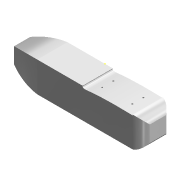
# Autodesk Inventor part: body
Saved by Autodesk Inventor 2020 (Build 240168000, 168)
## iProperties
Part Number: body
Material: Generic
Document SubType Name: Modeling
Designer: alifhabib
Appearance: Default
Author: alifhabib
Autodesk Inventor part; units mm, degrees
ref_plane "YZ Plane" through (0, 0, 0) normal (1, 0, 0) x (0, 1, 0)
ref_plane "XY Plane" through (0, 0, 0) normal (0, 0, 1) x (1, 0, 0)
sketch "Sketch1" plane through (0, 0, 0) normal (0, 0, 1) x (1, 0, 0)
  line L0 (-337.5, 75) -> (337.5, 75)
  line L1 (337.5, 75) -> (337.5, -75)
  line L2 (337.5, -75) -> (-337.5, -75)
  line L3 (-337.5, -75) -> (-337.5, 75)
  line L4 (-337.5, 75) -> (337.5, -75) construction
  line L5 (337.5, 75) -> (-337.5, -75) construction
  point P0 (0, 0)
  dimension "d0" = 675
  dimension "d1" = 150
  constraints: 12 end point, 2 midpoint, 2 parallel, 1 horizontal, 1 perpendicular
  measures "d0" distance of L1.end L2.end
  measures "d1" distance of L0.end L1.end
extrude "Extrusion1" add sketch "Sketch1" along normal blind 150
sketch "Sketch2" plane through (0, 0, 150) normal (0, 0, 1) x (1, 0, 0)
  line L0 (-400, 225) -> (400, 225)
  line L1 (400, 225) -> (400, -225)
  line L2 (400, -225) -> (-400, -225)
  line L3 (-400, -225) -> (-400, 225)
  line L4 (-337.5, 0) -> (-187.5, 0)
  line L5 (-337.5, 0) -> (-337.5, 40)
  line L6 (-337.5, 0) -> (-337.5, -40)
  line L7 (337.5, 0) -> (287.5, 0)
  line L8 (337.5, 0) -> (337.5, 40)
  line L9 (337.5, 0) -> (337.5, -40)
  arc A0 (-187.5, 75) -> (-337.5, 40) centre (-150.241, -423.6098) ccw
  line L10 (-187.5, 75) -> (287.5, 75)
  arc A1 (337.5, 40) -> (287.5, 75) centre (273.2116, 1.3736) ccw
  arc A2 (-337.5, -40) -> (-187.5, -75) centre (-150.241, 423.6098) ccw
  line L11 (-187.5, -75) -> (287.5, -75)
  arc A3 (287.5, -75) -> (337.5, -40) centre (273.2116, -1.3736) ccw
  point P0 (0, 0)
  dimension "d4" = 800
  dimension "d5" = 450
  dimension "d14" = 50
  dimension "d15" = 40
  dimension "d16" = 40
  dimension "d17" = 500
  dimension "d18" = 75
  constraints: 24 end point, 8 point on circle, 4 centre point, 4 symmetric about line, 3 horizontal, 2 parallel, 1 perpendicular, 2 other
  measures "d4" distance of L1.end L2.end
  measures "d5" distance of L0.end L1.end
  measures "d14" distance of L7.start L7.end
  measures "d15" distance of L7.start L8.end
  measures "d16" distance of L7.start L9.end
  measures "d17" radius of A0
  measures "d18" radius of A1
extrude "Extrusion2" cut sketch "Sketch2" against normal blind 150
sketch "Sketch3" plane through (-187.5, 75, 0) normal (0, 1, 0) x (1, 0, 0)
  line L0 (-312.5, 400) -> (687.5, 400)
  line L1 (687.5, 400) -> (687.5, -400)
  line L2 (687.5, -400) -> (-312.5, -400)
  line L3 (-312.5, -400) -> (-312.5, 400)
  line L4 (525, 0) -> (525, -150) projected
  line L5 (525, -75) -> (475, -75)
  line L6 (-150, -150) -> (-150, 0) projected
  line L7 (-150, -75) -> (-150, -35)
  line L8 (0, 0) -> (475, 0) projected
  arc A0 (0, 0) -> (-150, -35) centre (37.259, -498.6098) ccw
  line L9 (525, -75) -> (525, -35)
  line L10 (525, 0) -> (475, 0) projected
  arc A1 (525, -35) -> (475, 0) centre (460.7116, -73.6264) ccw
  line L11 (-150, -75) -> (-150, -115)
  arc A2 (-150, -115) -> (0, -150) centre (37.259, 348.6098) ccw
  line L12 (525, -75) -> (525, -115)
  arc A3 (475, -150) -> (525, -115) centre (460.7116, -76.3736) ccw
  line L13 (475, -150) -> (0, -150) projected
  line L14 (0, -150) -> (475, -150)
  point P0 (187.5, 0)
  dimension "d23" = 40
  dimension "d24" = 500
  dimension "d25" = 40
  dimension "d26" = 75
  constraints: 20 end point, 8 point on circle, 4 centre point, 2 horizontal, 2 midpoint, 2 parallel, 2 point on line, 1 perpendicular
  measures "d23" distance of L7.start L7.end
  measures "d24" radius of A0
  measures "d25" distance of L5.start L9.end
  measures "d26" radius of A1
extrude "Extrusion3" cut sketch "Sketch3" against normal blind 150 contours L0 L1 L2 L3 | L4 A1 L10
sketch "Sketch4" plane through (0, 0, 150) normal (0, 0, 1) x (1, 0, 0)
  spline S0 degree 4 poles (287.5, 72) (275.7106, 75.6696) (272.2633, 78.0977) (241.0041, 87.3899) (212.1922, 94.1056) (186.8012, 99.4436) (162.2405, 102.6617) (136.499, 103.3609) (115.3024, 103.9082) (87.5125, 99.0497) (77.8593, 96.7101) (62.5936, 91.6603) (56.4872, 88.8369) (50.2371, 85.9481) (43.0983, 79.8721) (41.263, 78.3038) (35.0709, 71.8313) (41.0621, 66.1136) (43.5349, 66.5804) (51.0426, 65.1949) (57.2037, 65.9223) (63.437, 66.335) (78.7454, 67.9836) (88.3716, 68.7088) (116.236, 70.8678) (137.1854, 71.569) (162.8258, 72.2403) (187.1936, 73.1117) (212.5281, 72.7462) (241.0177, 72.4966) (272.1667, 71.6209) (275.8592, 71.8531) (287.5, 71.2) knots 0 0 0 0 0 0.082908 0.121264 0.162409 0.203325 0.244067 0.284728 0.322462 0.357388 0.387441 0.412707 0.436373 0.45684 0.477222 0.496964 0.514702 0.533384 0.551956 0.570848 0.593257 0.617753 0.647324 0.681959 0.719554 0.76011 0.800663 0.841217 0.881776 0.91937 1 1 1 1 1
  arc A0 (287.5, 71.2) -> (287.5, 72) centre (286.5835, 71.6) ccw
  point P0 (0, 0)
  point P1 (274.89, 76.355)
  point P2 (262.2875, 80.71)
  point P3 (237.1175, 87.97)
  point P4 (211.975, 94.0325)
  point P5 (186.8575, 99.02)
  point P6 (161.785, 102.1575)
  point P7 (136.7575, 103.3225)
  point P8 (111.775, 102.5875)
  point P9 (86.8675, 98.68)
  point P10 (74.4425, 95.465)
  point P11 (62.0425, 91.2)
  point P12 (55.855, 88.53)
  point P13 (49.685, 85.06)
  point P14 (43.5475, 80.2425)
  point P15 (40.49, 77.395)
  point P16 (37.5, 71.6)
  point P17 (40.73, 67.15)
  point P18 (43.875, 66.3)
  point P19 (50.14, 65.645)
  point P20 (56.385, 65.7925)
  point P21 (62.6225, 66.3375)
  point P22 (75.095, 67.555)
  point P23 (87.57, 68.6475)
  point P24 (112.5275, 70.43)
  point P25 (137.5025, 71.54)
  point P26 (162.485, 72.275)
  point P27 (187.47, 72.86)
  point P28 (212.4725, 72.77)
  point P29 (237.48, 72.43)
  point P30 (262.4925, 71.94)
  point P31 (274.9975, 71.7075)
  point P32 (287.5, 75)
  dimension "d31" = 1
  constraints: 2 point on circle, 1 centre point, 33 other
  measures "d31" radius of A0
extrude "Extrusion4" cut sketch "Sketch4" against normal blind 150
sketch "Sketch5" plane through (0, 0, 150) normal (0, 0, 1) x (1, 0, 0)
  spline S0 degree 4 poles (278.5919, 75) (280.4602, 74.3245) (282.4435, 73.6259) (284.707, 72.8694) (287.5, 72) knots 0 0 0 0 0 1 1 1 1 1 projected
  line L0 (287.5, 72) -> (287.5, 75) projected
  line L1 (287.5, 75) -> (278.5919, 75) projected
  point P0 (0, 0)
  constraints: 1 other
extrude "Extrusion5" cut sketch "Sketch5" against normal blind 150
sketch "Sketch8" plane through (0, 0, 150) normal (0, 0, 1) x (1, 0, 0)
  line L0 (38.5386, 75) -> (-187.5, 75) projected
  line L1 (-187.5, 75) -> (-187.5, -75) projected
  line L2 (-187.5, -75) -> (287.5, -75) projected
  line L3 (287.5, -75) -> (287.5, 71.2) projected
  arc A0 (-337.5, -40) -> (-187.5, -75) centre (-150.241, 423.6098) ccw projected
  line L4 (-187.5, 75) -> (-187.5, -75) projected
  arc A1 (-187.5, 75) -> (-337.5, 40) centre (-150.241, -423.6098) ccw projected
  line L5 (-337.5, -40) -> (-337.5, 40) projected
  line L6 (287.5, -75) -> (287.5, 71.2) projected
  arc A2 (287.5, -75) -> (337.5, -40) centre (273.2116, -1.3736) ccw projected
  line L7 (337.5, 40) -> (337.5, -40) projected
  arc A3 (337.5, 40) -> (287.5, 75) centre (273.2116, 1.3736) ccw projected
  line L8 (287.5, 72) -> (287.5, 75) projected
  point P0 (0, 0)
  constraints: 1 vertical alignment, 1 other
sketch "Sketch9" plane through (-187.5, 75, 150) normal (0, 1, 0) x (1, 0, 0)
  point P0 (187.5, 150)
sketch "Sketch10" plane through (-337.5, -40, 115) normal (-1, 0, 0) x (0, 0, 1)
  line L0 (0, 0) -> (0, 80) projected
  line L1 (0, 80) -> (-80, 80) projected
  line L2 (-80, 80) -> (-80, 0) projected
  line L3 (-80, 0) -> (0, 0) projected
  point P0 (-115, 40)
ref_plane "Work Plane1" through (0, 60, 0) normal (0, 1, 0) x (-1, 0, 0)
sketch "Sketch11" plane through (0, 60, 0) normal (0, 1, 0) x (-1, 0, 0)
  line L0 (-287.5, 0) -> (-287.5, 150) projected
  line L1 (-287.5, 75) -> (-287.5, 47.5)
  line L2 (-287.5, 47.5) -> (-237.5, 47.5)
  circle A0 centre (-237.5, 47.5) radius 4
  line L3 (-287.5, 75) -> (-187.5, 75)
  line L4 (-287.5, 47.5) -> (-87.5, 47.5)
  circle A1 centre (-87.5, 47.5) radius 4
  circle A2 centre (-237.5, 102.5) radius 4
  circle A3 centre (-87.5, 102.5) radius 4
  point P0 (0, 0)
  dimension "d70" = 27.5
  dimension "d71" = 50
  dimension "d72" = 8
  dimension "d73" = 100
  dimension "d74" = 200
  dimension "d75" = 8
  constraints: 8 end point, 4 centre point, 4 coincident, 4 symmetric about line, 2 horizontal, 2 point on line, 1 midpoint, 2 other
  measures "d70" distance of L1.start L1.end
  measures "d71" distance of L1.end L2.end
  measures "d72" diameter of A0
  measures "d73" distance of L1.start L3.end
  measures "d74" distance of L1.end L4.end
  measures "d75" diameter of A1
extrude "Extrusion8" cut sketch "Sketch11" against normal mid plane 100
body "Solid1"
